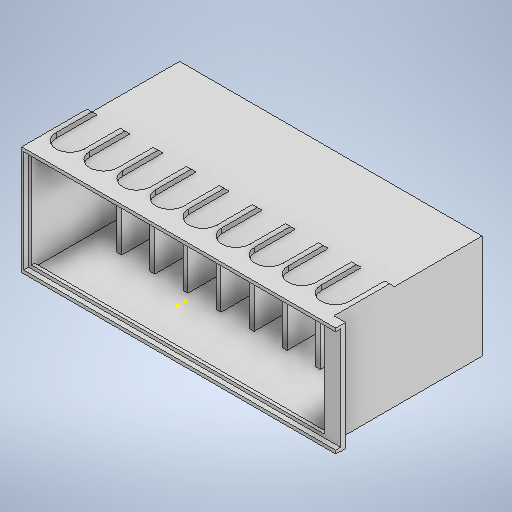
# Autodesk Inventor part: Storage
Saved by Autodesk Inventor 2025.2 (Build 292293000, 293)
## iProperties
Created: 2025-04-05
Part Number: Storage
Material: Generic
Document SubType Name: Modeling
Designer: pipep
Density: 1 g/cm^3
Appearance: Default
Author: pipep
Autodesk Inventor part; units mm, degrees
ref_plane "YZ Plane" through (0, 0, 0) normal (1, 0, 0) x (0, 1, 0)
ref_plane "XZ Plane" through (0, 0, 0) normal (0, 1, 0) x (-1, 0, 0)
ref_plane "XY Plane" through (0, 0, 0) normal (0, 0, 1) x (1, 0, 0)
sketch "Sketch1" plane through (0, 0, 0) normal (0, 0, 1) x (1, 0, 0)
  line L0 (2.6533, -0.0823) -> (-97.3467, -0.0823)
  line L1 (-97.3467, -0.0823) -> (-97.3467, 31.7677)
  line L2 (-97.3467, 31.7677) -> (102.6533, 31.7677)
  line L3 (102.6533, 31.7677) -> (102.6533, -31.9323)
  line L4 (102.6533, -31.9323) -> (-97.3467, -31.9323)
  line L5 (-97.3467, -31.9323) -> (-97.3467, 31.7677)
  point P0 (0, 0)
  dimension "d0" = 100
  dimension "d1" = 31.85
  dimension "d2" = 200
  dimension "d3" = 63.7
  constraints: 12 end point, 2 horizontal, 2 parallel, 2 perpendicular
  measures "d0" distance of L0.start L0.end
  measures "d1" distance of L0.end L1.end
  measures "d2" distance of L3.end L4.end
  measures "d3" distance of L2.end L3.end
extrude "Extrusion1" add sketch "Sketch1" along normal blind 56.62
sketch "Sketch2" plane through (0, 0, 56.62) normal (0, 0, 1) x (1, 0, 0)
  line L0 (-97.3467, 31.7677) -> (-97.3467, -31.9323) projected
  line L1 (-97.3467, -0.0823) -> (-94.3467, -0.0823)
  line L2 (-94.3467, -0.0823) -> (-94.3467, 29.7677)
  line L3 (-94.3467, 29.7677) -> (-77.1067, 29.7677)
  line L4 (102.6533, 31.7677) -> (-97.3467, 31.7677) projected
  line L5 (-94.3467, 29.7677) -> (-77.1067, 29.7677)
  line L6 (-77.1067, 29.7677) -> (-77.1067, -29.9323)
  line L7 (-77.1067, -29.9323) -> (-94.3467, -29.9323)
  line L8 (-94.3467, -29.9323) -> (-94.3467, 29.7677)
  line L9 (-77.1067, -0.0823) -> (-74.1067, -0.0823)
  line L10 (-74.1067, -0.0823) -> (-74.1067, 29.7677)
  line L11 (-74.1067, 29.7677) -> (-56.8667, 29.7677)
  line L12 (-74.1067, 29.7677) -> (-56.8667, 29.7677)
  line L13 (-56.8667, 29.7677) -> (-56.8667, -29.9323)
  line L14 (-56.8667, -29.9323) -> (-74.1067, -29.9323)
  line L15 (-74.1067, -29.9323) -> (-74.1067, 29.7677)
  line L16 (-56.8667, -0.0823) -> (-53.8667, -0.0823)
  line L17 (-53.8667, -0.0823) -> (-53.8667, 29.7677)
  line L18 (-53.8667, 29.7677) -> (-36.6267, 29.7677)
  line L19 (-53.8667, 29.7677) -> (-36.6267, 29.7677)
  line L20 (-36.6267, 29.7677) -> (-36.6267, -29.9323)
  line L21 (-36.6267, -29.9323) -> (-53.8667, -29.9323)
  line L22 (-53.8667, -29.9323) -> (-53.8667, 29.7677)
  line L23 (-36.6267, -0.0823) -> (-33.6267, -0.0823)
  line L24 (-33.6267, -0.0823) -> (-33.6267, 29.7677)
  line L25 (-33.6267, 29.7677) -> (-16.3867, 29.7677)
  line L26 (-33.6267, 29.7677) -> (-16.3867, 29.7677)
  line L27 (-16.3867, 29.7677) -> (-16.3867, -29.9323)
  line L28 (-16.3867, -29.9323) -> (-33.6267, -29.9323)
  line L29 (-33.6267, -29.9323) -> (-33.6267, 29.7677)
  line L30 (-16.3867, -0.0823) -> (-13.3867, -0.0823)
  line L31 (-13.3867, -0.0823) -> (-13.3867, 29.7677)
  line L32 (-13.3867, 29.7677) -> (3.8533, 29.7677)
  line L33 (-13.3867, 29.7677) -> (3.8533, 29.7677)
  line L34 (3.8533, 29.7677) -> (3.8533, -29.9323)
  line L35 (3.8533, -29.9323) -> (-13.3867, -29.9323)
  line L36 (-13.3867, -29.9323) -> (-13.3867, 29.7677)
  line L37 (3.8533, -0.0823) -> (6.8533, -0.0823)
  line L38 (6.8533, -0.0823) -> (6.8533, 29.7677)
  line L39 (6.8533, 29.7677) -> (24.0933, 29.7677)
  line L40 (6.8533, 29.7677) -> (24.0933, 29.7677)
  line L41 (24.0933, 29.7677) -> (24.0933, -29.9323)
  line L42 (24.0933, -29.9323) -> (6.8533, -29.9323)
  line L43 (6.8533, -29.9323) -> (6.8533, 29.7677)
  line L44 (24.0933, -0.0823) -> (27.0933, -0.0823)
  line L45 (27.0933, -0.0823) -> (27.0933, 29.7677)
  line L46 (27.0933, 29.7677) -> (44.3333, 29.7677)
  line L47 (27.0933, 29.7677) -> (44.3333, 29.7677)
  line L48 (44.3333, 29.7677) -> (44.3333, -29.9323)
  line L49 (44.3333, -29.9323) -> (27.0933, -29.9323)
  line L50 (27.0933, -29.9323) -> (27.0933, 29.7677)
  line L51 (64.5733, -0.0823) -> (67.5733, -0.0823)
  line L52 (67.5733, -0.0823) -> (67.5733, 29.7677)
  line L53 (67.5733, 29.7677) -> (84.8133, 29.7677)
  line L54 (67.5733, 29.7677) -> (84.8133, 29.7677)
  line L55 (84.8133, 29.7677) -> (84.8133, -29.9323)
  line L56 (84.8133, -29.9323) -> (67.5733, -29.9323)
  line L57 (67.5733, -29.9323) -> (67.5733, 29.7677)
  line L58 (84.8133, -0.0823) -> (87.8133, -0.0823)
  line L59 (87.8133, -0.0823) -> (87.8133, 29.7677)
  line L60 (87.8133, 29.7677) -> (105.0533, 29.7677)
  line L61 (87.8133, 29.7677) -> (105.0533, 29.7677)
  line L62 (105.0533, 29.7677) -> (105.0533, -29.9323)
  line L63 (105.0533, -29.9323) -> (87.8133, -29.9323)
  line L64 (87.8133, -29.9323) -> (87.8133, 29.7677)
  line L65 (44.3333, -0.0823) -> (47.3333, -0.0823)
  line L66 (47.3333, -0.0823) -> (47.3333, 29.7677)
  line L67 (47.3333, 29.7677) -> (64.5733, 29.7677)
  line L68 (47.3333, 29.7677) -> (64.5733, 29.7677)
  line L69 (64.5733, 29.7677) -> (64.5733, -29.9323)
  line L70 (64.5733, -29.9323) -> (47.3333, -29.9323)
  line L71 (47.3333, -29.9323) -> (47.3333, 29.7677)
  line L72 (87.8133, -35.0469) -> (105.0533, -35.0469)
  line L73 (105.0533, -35.0469) -> (105.0533, 39.0477)
  line L74 (105.0533, 39.0477) -> (87.8133, 39.0477)
  line L75 (87.8133, 39.0477) -> (87.8133, -35.0469)
  point P0 (0, 0)
  dimension "d6" = 3
  dimension "d7" = 29.85
  dimension "d8" = 17.24
  dimension "d9" = 90
  dimension "d10" = 59.7
  dimension "d11" = 3
  dimension "d12" = 29.85
  dimension "d13" = 17.24
  dimension "d14" = 90
  dimension "d15" = 59.7
  dimension "d16" = 3
  dimension "d17" = 29.85
  dimension "d18" = 17.24
  dimension "d19" = 90
  dimension "d20" = 59.7
  dimension "d21" = 3
  dimension "d22" = 29.85
  dimension "d23" = 17.24
  dimension "d24" = 90
  dimension "d25" = 59.7
  dimension "d26" = 3
  dimension "d27" = 29.85
  dimension "d28" = 17.24
  dimension "d29" = 90
  dimension "d30" = 59.7
  dimension "d31" = 3
  dimension "d32" = 29.85
  dimension "d33" = 17.24
  dimension "d34" = 90
  dimension "d35" = 59.7
  dimension "d36" = 3
  dimension "d37" = 29.85
  dimension "d38" = 17.24
  dimension "d39" = 90
  dimension "d40" = 59.7
  dimension "d41" = 3
  dimension "d42" = 29.85
  dimension "d43" = 17.24
  dimension "d44" = 90
  dimension "d45" = 59.7
  dimension "d46" = 3
  dimension "d47" = 29.85
  dimension "d48" = 17.24
  dimension "d49" = 90
  dimension "d50" = 59.7
  dimension "d51" = 3
  dimension "d52" = 29.85
  dimension "d53" = 17.24
  dimension "d54" = 90
  dimension "d55" = 59.7
  constraints: 148 end point, 23 parallel, 21 horizontal, 21 perpendicular, 1 midpoint
  measures "d6" distance of L1.start L1.end
  measures "d7" distance of L1.end L2.end
  measures "d8" distance of L2.end L3.end
  measures "d9" angle of L2 L3
  measures "d10" distance of L5.end L6.end
  measures "d11" distance of L9.start L9.end
  measures "d12" distance of L9.end L10.end
  measures "d13" distance of L10.end L11.end
  measures "d14" angle of L10 L11
  measures "d15" distance of L12.end L13.end
  measures "d16" distance of L16.start L16.end
  measures "d17" distance of L16.end L17.end
  measures "d18" distance of L17.end L18.end
  measures "d19" angle of L17 L18
  measures "d20" distance of L19.end L20.end
  measures "d21" distance of L23.start L23.end
  measures "d22" distance of L23.end L24.end
  measures "d23" distance of L24.end L25.end
  measures "d24" angle of L24 L25
  measures "d25" distance of L26.end L27.end
  measures "d26" distance of L30.start L30.end
  measures "d27" distance of L30.end L31.end
  measures "d28" distance of L31.end L32.end
  measures "d29" angle of L31 L32
  measures "d30" distance of L33.end L34.end
  measures "d31" distance of L37.start L37.end
  measures "d32" distance of L37.end L38.end
  measures "d33" distance of L38.end L39.end
  measures "d34" angle of L38 L39
  measures "d35" distance of L40.end L41.end
  measures "d36" distance of L44.start L44.end
  measures "d37" distance of L44.end L45.end
  measures "d38" distance of L45.end L46.end
  measures "d39" angle of L45 L46
  measures "d40" distance of L47.end L48.end
  measures "d41" distance of L51.start L51.end
  measures "d42" distance of L51.end L52.end
  measures "d43" distance of L52.end L53.end
  measures "d44" angle of L52 L53
  measures "d45" distance of L54.end L55.end
  measures "d46" distance of L58.start L58.end
  measures "d47" distance of L58.end L59.end
  measures "d48" distance of L59.end L60.end
  measures "d49" angle of L59 L60
  measures "d50" distance of L61.end L62.end
  measures "d51" distance of L65.start L65.end
  measures "d52" distance of L65.end L66.end
  measures "d53" distance of L66.end L67.end
  measures "d54" angle of L66 L67
  measures "d55" distance of L68.end L69.end
extrude "Extrusion2" cut sketch "Sketch2" against normal blind 56.62 contours L75 L74 L73 L60 | L2 L3 L6 L7 L8 | L60 L62 L63 L64 L59 | L55 L56 L57 L52 L53 | L63 L73 L72 L75 | L10 L11 L13 L14 L15 | L69 L70 L71 L66 L67 | L17 L18 L20 L21 L22 | L48 L49 L50 L45 L46 | L24 L25 L27 L28 L29 | L41 L42 L43 L38 L39 | L31 L32 L34 L35 L36
sketch "Sketch4" plane through (0, 0, 0) normal (0, 0, -1) x (-1, 0, 0)
  line L0 (-87.8133, 31.7677) -> (-87.8133, -31.9323) projected
  line L1 (97.3467, -31.9323) -> (-87.8133, -31.9323) projected
  line L2 (-87.8133, 31.7677) -> (97.3467, 31.7677)
  line L3 (97.3467, 31.7677) -> (97.3467, -31.9323)
  line L4 (97.3467, -31.9323) -> (-87.8133, -31.9323)
  line L5 (-87.8133, -31.9323) -> (-87.8133, 31.7677)
  point P0 (0, 0)
  constraints: 8 end point, 2 parallel, 1 horizontal, 1 perpendicular
extrude "Extrusion4" add sketch "Sketch4" along normal blind 2
sketch "Sketch5" plane through (0, 0, 56.62) normal (0, 0, 1) x (1, 0, 0)
  line L0 (-94.3467, 29.7677) -> (-94.3467, 34.7677)
  line L1 (-94.3467, 34.7677) -> (-97.3467, 34.7677)
  line L2 (-97.3467, 34.7677) -> (87.8133, 34.7677)
  line L3 (87.8133, 34.7677) -> (87.8133, -31.9323)
  line L4 (87.8133, -31.9323) -> (-97.3467, -31.9323)
  line L5 (-97.3467, -31.9323) -> (-97.3467, 34.7677)
  line L6 (84.8133, 29.7677) -> (84.8133, -29.9323) projected
  line L7 (-94.3467, 29.7677) -> (84.8133, 29.7677)
  line L8 (84.8133, 29.7677) -> (84.8133, -29.9323)
  line L9 (84.8133, -29.9323) -> (-94.3467, -29.9323)
  line L10 (-94.3467, -29.9323) -> (-94.3467, 29.7677)
  point P0 (0, 0)
  dimension "d69" = 5
  dimension "d70" = 3
  constraints: 20 end point, 4 parallel, 3 horizontal, 2 perpendicular, 1 vertical
  measures "d69" distance of L0.start L0.end
  measures "d70" distance of L0.end L1.end
extrude "Extrusion5" add sketch "Sketch5" along normal blind 40 and the other way blind 5
sketch "Sketch11" plane through (87.8133, -31.9323, -2) normal (1, 0, 0) x (0, 0, -1)
  line L0 (-98.62, 66.7) -> (-53.62, 66.7) projected
  line L1 (-98.62, 66.7) -> (-98.62, 64.7)
  line L2 (-98.62, 66.7) -> (-98.62, 0) projected
  line L3 (-98.62, 64.7) -> (-93.62, 64.7)
  line L4 (-98.62, 0) -> (-98.62, 2.6466)
  line L5 (0, 0) -> (-98.62, 0) projected
  line L6 (-98.62, 2) -> (-98.62, 61.7) projected
  line L7 (-98.62, 0) -> (-98.62, 2)
  line L8 (-98.62, 2) -> (-96.62, 2)
  line L9 (-93.62, 64.7) -> (-96.62, 64.7)
  line L10 (-96.62, 64.7) -> (-96.62, 2)
  line L11 (-96.62, 2) -> (-93.62, 2)
  line L12 (-93.62, 2) -> (-93.62, 64.7)
  point P0 (-2, 31.9323)
  dimension "d95" = 2
  dimension "d96" = 5
  dimension "d97" = 2
  dimension "d98" = 2
  constraints: 18 end point, 2 horizontal, 2 parallel, 2 perpendicular, 2 point on line, 1 vertical
  measures "d95" distance of L0.start L1.end
  measures "d96" distance of L1.end L3.end
  measures "d97" distance of L2.end L6.start
  measures "d98" distance of L6.start L8.end
extrude "Extrusion10" cut sketch "Sketch11" against normal blind 184 contours L3 L12 L11 L10
sketch "Sketch12" plane through (-94.3467, -29.9323, 96.62) normal (1, 0, 0) x (0, 0, -1)
  line L0 (0, 0) -> (2, 0) projected
  line L1 (0, 0) -> (0, 3)
  line L2 (0, 0) -> (0, 59.7) projected
  line L3 (0, 3) -> (2, 3)
  line L4 (2, 3) -> (2, 0)
  line L5 (2, 0) -> (0, 0)
  line L6 (5, 0) -> (5, 3)
  line L7 (5, 59.7) -> (5, 0) projected
  line L8 (5, 3) -> (7, 3)
  line L9 (7, 3) -> (7, 0)
  line L10 (5, 0) -> (96.62, 0) projected
  line L11 (7, 0) -> (5, 0)
  point P0 (96.62, 29.9323)
  dimension "d101" = 3
  dimension "d102" = 2
  dimension "d103" = 3
  dimension "d104" = 3
  dimension "d105" = 2
  dimension "d106" = 3
  dimension "d107" = 2
  constraints: 16 end point, 4 point on line, 2 perpendicular
  measures "d101" distance of L0.start L1.end
  measures "d102" distance of L1.end L3.end
  measures "d103" distance of L3.end L4.end
  measures "d104" distance of L6.start L6.end
  measures "d105" distance of L6.end L8.end
  measures "d106" distance of L8.end L9.end
  measures "d107" distance of L9.end L6.start
extrude "Extrusion11" add sketch "Sketch12" along normal blind 180
sketch "Sketch13" plane through (0, 0, 96.62) normal (0, 0, 1) x (1, 0, 0)
  point P0 (0, 0)
sketch "Sketch14" plane through (87.8133, -29.9323, 91.62) normal (0, 0, 1) x (1, 0, 0)
  point P0 (-87.8133, 29.9323)
sketch "Sketch15" plane through (0, 0, 96.62) normal (0, 0, 1) x (1, 0, 0)
  line L0 (87.8133, 34.7677) -> (-97.3467, 34.7677) projected
  line L1 (87.8133, -31.9323) -> (87.8133, 34.7677) projected
  line L2 (-97.3467, 34.7677) -> (87.8133, 34.7677)
  line L3 (87.8133, 34.7677) -> (87.8133, -31.9323)
  line L4 (87.8133, -31.9323) -> (-97.3467, -31.9323)
  line L5 (-97.3467, -31.9323) -> (-97.3467, 34.7677)
  point P0 (0, 0)
  constraints: 8 end point, 2 parallel, 1 horizontal, 1 perpendicular
extrude "Extrusion12" cut sketch "Sketch15" against normal blind 2
sketch "Sketch16" plane through (0, 0, 0) normal (0, 0, 1) x (1, 0, 0)
  point P0 (0, 0)
sketch "Sketch17" plane through (-94.3467, -26.9323, 89.62) normal (0, 1, 0) x (1, 0, 0)
  line L0 (0, 0) -> (179.16, 0) projected
  line L1 (0, 0) -> (179.16, 0)
  line L2 (179.16, 0) -> (179.16, -2)
  line L3 (179.16, -2) -> (0, -2)
  line L4 (0, -2) -> (0, 0)
  point P0 (94.3467, 89.62)
  constraints: 8 end point, 2 parallel, 1 horizontal, 1 perpendicular
extrude "Extrusion13" cut sketch "Sketch17" against normal blind 1
sketch "Sketch18" plane through (-97.3467, 34.7677, 51.62) normal (0, 1, 0) x (1, 0, 0)
  line L0 (185.16, 0) -> (182.16, 0)
  line L1 (0, -43) -> (0, 0) projected
  line L2 (0, 0) -> (3, 0)
  line L3 (3, -40) -> (3, 51.62) projected
  line L4 (3, 0) -> (3, -25)
  line L5 (185.16, -43) -> (1.16, -43) projected
  arc A0 (3, -25) -> (20.24, -25) centre (11.62, -25) ccw
  line L6 (3, 0) -> (20.24, 0)
  line L7 (20.24, 0) -> (20.24, -25)
  line L8 (3, -25) -> (3, 0)
  line L9 (23.24, 0.3271) -> (23.24, -24.6729)
  arc A1 (23.24, -24.6729) -> (40.48, -24.6729) centre (31.86, -24.6729) ccw
  line L10 (40.48, 0.3271) -> (40.48, -24.6729)
  line L11 (23.24, -24.6729) -> (23.24, 0.3271)
  line L12 (43.48, 0.3271) -> (43.48, -24.6729)
  arc A2 (43.48, -24.6729) -> (60.72, -24.6729) centre (52.1, -24.6729) ccw
  line L13 (60.72, 0.3271) -> (60.72, -24.6729)
  line L14 (43.48, -24.6729) -> (43.48, 0.3271)
  line L15 (63.72, 0.3271) -> (63.72, -24.6729)
  arc A3 (63.72, -24.6729) -> (80.96, -24.6729) centre (72.34, -24.6729) ccw
  line L16 (80.96, 0.3271) -> (80.96, -24.6729)
  line L17 (63.72, -24.6729) -> (63.72, 0.3271)
  line L18 (83.96, 0.3271) -> (83.96, -24.6729)
  arc A4 (83.96, -24.6729) -> (101.2, -24.6729) centre (92.58, -24.6729) ccw
  line L19 (101.2, 0.3271) -> (101.2, -24.6729)
  line L20 (83.96, -24.6729) -> (83.96, 0.3271)
  line L21 (104.2, 0.3271) -> (104.2, -24.6729)
  arc A5 (104.2, -24.6729) -> (121.44, -24.6729) centre (112.82, -24.6729) ccw
  line L22 (121.44, 0.3271) -> (121.44, -24.6729)
  line L23 (104.2, -24.6729) -> (104.2, 0.3271)
  line L24 (124.44, 0.3271) -> (124.44, -24.6729)
  arc A6 (124.44, -24.6729) -> (141.68, -24.6729) centre (133.06, -24.6729) ccw
  line L25 (141.68, 0.3271) -> (141.68, -24.6729)
  line L26 (124.44, -24.6729) -> (124.44, 0.3271)
  line L27 (144.68, 0.3271) -> (144.68, -24.6729)
  arc A7 (144.68, -24.6729) -> (161.92, -24.6729) centre (153.3, -24.6729) ccw
  line L28 (161.92, 0.3271) -> (161.92, -24.6729)
  line L29 (144.68, -24.6729) -> (144.68, 0.3271)
  line L30 (164.92, 0.3271) -> (164.92, -24.6729)
  arc A8 (164.92, -24.6729) -> (182.16, -24.6729) centre (173.54, -24.6729) ccw
  line L31 (182.16, 0) -> (182.16, -24.6729)
  line L32 (164.92, -24.6729) -> (164.92, 0.3271)
  line L33 (20.24, 0) -> (182.16, 0)
  line L34 (0, 0) -> (185.16, 0) projected
  point P0 (97.3467, 51.62)
  point P1 (3, -25)
  point P2 (161.92, 0)
  point P3 (144.68, 0)
  point P4 (40.48, 0)
  point P5 (23.24, 0)
  point P6 (141.68, 0)
  point P7 (124.44, 0)
  point P8 (60.72, 0)
  point P9 (43.48, 0)
  point P10 (121.44, 0)
  point P11 (104.2, 0)
  point P12 (80.96, 0)
  point P13 (63.72, 0)
  point P14 (101.2, 0)
  point P15 (83.96, 0)
  point P16 (164.92, 0)
  dimension "d115" = 3
  dimension "d119" = 3
  dimension "d120" = 25
  dimension "d121" = 17.24
  dimension "d122" = 25
  dimension "d123" = 17.24
  dimension "d124" = 25
  dimension "d125" = 17.24
  dimension "d126" = 25
  dimension "d127" = 17.24
  dimension "d128" = 25
  dimension "d129" = 17.24
  dimension "d130" = 25
  dimension "d131" = 17.24
  dimension "d132" = 25
  dimension "d133" = 17.24
  dimension "d134" = 25
  dimension "d135" = 17.24
  dimension "d138" = 25
  dimension "d139" = 17.24
  constraints: 62 end point, 18 point on circle, 9 centre point, 9 parallel, 9 tangent, 2 perpendicular, 1 collinear, 1 horizontal, 1 point on line
  measures "d115" distance of L0.start L0.end
  measures "d119" distance of L1.end L2.end
  measures "d120" distance of L2.end L4.end
  measures "d121" distance of L4.end L7.end
  measures "d122" distance of L9.start L9.end
  measures "d123" distance of L9.end L10.end
  measures "d124" distance of L12.start L12.end
  measures "d125" distance of L12.end L13.end
  measures "d126" distance of L15.start L15.end
  measures "d127" distance of L15.end L16.end
  measures "d128" distance of L18.start L18.end
  measures "d129" distance of L18.end L19.end
  measures "d130" distance of L21.start L21.end
  measures "d131" distance of L21.end L22.end
  measures "d132" distance of L24.start L24.end
  measures "d133" distance of L24.end L25.end
  measures "d134" distance of L27.start L27.end
  measures "d135" distance of L27.end L28.end
  measures "d138" distance of L30.start L30.end
  measures "d139" distance of L30.end L31.end
extrude "Extrusion14" cut sketch "Sketch18" against normal blind 3
chamfer "Chamfer1" distance 3 angle 45 10 edges at (-95.8467, 34.7677, 51.62) (-75.6067, 34.7677, 51.62) (-55.3667, 34.7677, 51.62) (-35.1267, 34.7677, 51.62) (-14.8867, 34.7677, 51.62) (5.3533, 34.7677, 51.62) (25.5933, 34.7677, 51.62) (45.8333, 34.7677, 51.62) (66.0733, 34.7677, 51.62) (86.3133, 34.7677, 51.62)
sketch "Sketch19" plane through (-94.3467, 29.7677, 0) normal (0, -1, 0) x (1, 0, 0)
  point P0 (94.3467, 0)
sketch "Sketch20" plane through (-94.3467, 29.7677, 0) normal (0, -1, 0) x (1, 0, 0)
  point P0 (94.3467, 0)
sketch "Sketch21" plane through (0, 0, -2) normal (0, 0, -1) x (-1, 0, 0)
  point P0 (0, 0)
sketch "Sketch22" plane through (87.8133, -31.9323, -2) normal (1, 0, 0) x (0, 0, -1)
  line L0 (0, 0) -> (-96.62, 0)
  line L1 (-96.62, 66.7) -> (-56.62, 66.7) projected
  line L2 (-96.62, 0) -> (-96.62, 66.7)
  line L3 (-96.62, 66.7) -> (-93.62, 66.7)
  line L4 (-93.62, 66.7) -> (-93.62, 0)
  line L5 (-96.62, 66.7) -> (-93.62, 66.7)
  line L6 (-93.62, 66.7) -> (-93.62, 64.7)
  line L7 (-93.62, 64.7) -> (-96.62, 64.7)
  line L8 (-96.62, 64.7) -> (-96.62, 66.7)
  line L9 (-96.62, 0) -> (-93.62, 0)
  line L10 (-93.62, 0) -> (-93.62, 2)
  line L11 (-93.62, 2) -> (-96.62, 2)
  line L12 (-96.62, 2) -> (-96.62, 0)
  line L13 (-93.62, 66.7) -> (-90.62, 66.7)
  line L14 (-90.62, 66.7) -> (-90.62, -0.2532)
  line L15 (-90.62, -0.2532) -> (-93.62, -0.2532)
  line L16 (-93.62, -0.2532) -> (-93.62, 66.7)
  point P0 (-2, 31.9323)
  point P1 (-93.62, 2)
  point P2 (-96.62, 2)
  dimension "d148" = 3
  dimension "d149" = 3
  dimension "d150" = 2
  dimension "d151" = 3
  dimension "d152" = 2
  dimension "d153" = 3
  constraints: 32 end point, 6 parallel, 5 perpendicular, 3 horizontal, 2 point on line
  measures "d148" distance of L1.start L3.end
  measures "d149" distance of L6.end L7.end
  measures "d150" distance of L5.end L6.end
  measures "d151" distance of L11.end L10.end
  measures "d152" distance of L10.end L9.end
  measures "d153" distance of L14.end L15.end
extrude "Extrusion15" add sketch "Sketch22" along normal blind 7 contours L4 L1 L14 L0 | L0 L2 L11 L4 | L0 L14 L15 L16 | L7 L2 L1 L4
sketch "Sketch6" plane through (87.8133, -31.9323, -2) normal (1, 0, 0) x (0, 0, -1)
  line L0 (-98.62, 0) -> (-98.62, 66.7) projected
  line L1 (-98.62, 66.7) -> (-98.62, 64.7)
  line L2 (-98.62, 64.7) -> (-93.62, 64.7)
  line L3 (-98.62, 0) -> (0, 0) projected
  line L4 (-98.62, 0) -> (-98.62, 2)
  line L5 (-98.62, 2) -> (-96.62, 2)
  line L6 (-93.62, 64.7) -> (-96.62, 64.7)
  line L7 (-96.62, 64.7) -> (-96.62, 2)
  line L8 (-96.62, 2) -> (-93.62, 2)
  line L9 (-93.62, 2) -> (-93.62, 64.7)
  point P0 (-2, 31.9323)
  dimension "d75" = 2
  dimension "d76" = 5
  dimension "d77" = 2
  dimension "d78" = 2
  constraints: 16 end point, 3 perpendicular, 2 parallel, 2 point on line, 1 horizontal
  measures "d75" distance of L0.end L1.end
  measures "d76" distance of L1.end L2.end
  measures "d77" distance of L0.start L4.end
  measures "d78" distance of L4.end L5.end
sketch "Sketch7" plane through (-94.3467, -29.9323, 96.62) normal (1, 0, 0) x (0, 0, -1)
  line L0 (0, 0) -> (0, 3)
  line L1 (0, 0) -> (0, 59.7) projected
  line L2 (0, 3) -> (2, 3)
  line L3 (2, 3) -> (2, 0)
  line L4 (2, 0) -> (0, 0)
  line L5 (5, 59.7) -> (5, 0) projected
  line L6 (5, 0) -> (5, 3)
  line L7 (5, 3) -> (7, 3)
  line L8 (7, 3) -> (7, 0)
  line L9 (7, 0) -> (5, 0)
  point P0 (96.62, 29.9323)
  dimension "d81" = 3
  dimension "d82" = 2
  dimension "d83" = 3
  dimension "d84" = 2
  dimension "d85" = 3
  constraints: 16 end point, 4 point on line, 3 perpendicular
  measures "d81" distance of L0.start L0.end
  measures "d82" distance of L0.end L2.end
  measures "d83" distance of L5.end L6.end
  measures "d84" distance of L6.end L7.end
  measures "d85" distance of L7.end L8.end
sketch "Sketch8" plane through (0, 0, 96.62) normal (0, 0, 1) x (1, 0, 0)
  line L0 (87.8133, 34.7677) -> (-97.3467, 34.7677) projected
  line L1 (-97.3467, 34.7677) -> (-97.3467, 36.7677)
  line L2 (87.8133, 34.7677) -> (87.8133, 36.7677)
  line L3 (-97.3467, 36.7677) -> (87.8133, 36.7677)
  line L4 (-97.3467, -31.9323) -> (87.8133, -31.9323) projected
  line L5 (-97.3467, 34.7677) -> (87.8133, 34.7677)
  line L6 (87.8133, 34.7677) -> (87.8133, -31.9323)
  line L7 (87.8133, -31.9323) -> (-97.3467, -31.9323)
  line L8 (-97.3467, -31.9323) -> (-97.3467, 34.7677)
  point P0 (0, 0)
  dimension "d88" = 2
  dimension "d89" = 2
  dimension "d90" = 185.16
  constraints: 14 end point, 2 parallel, 2 vertical, 1 horizontal, 1 perpendicular
  measures "d88" distance of L0.end L1.end
  measures "d89" distance of L0.start L2.end
  measures "d90" distance of L1.end L2.end
sketch "Sketch9" plane through (87.8133, -29.9323, 91.62) normal (0, 0, 1) x (1, 0, 0)
  line L0 (-3, 0) -> (-3, 3) projected
  line L1 (0, 0) -> (-3, 0)
  line L2 (-3, 0) -> (-3, 3)
  line L3 (-3, 3) -> (0, 3)
  line L4 (0, 3) -> (0, 0)
  line L5 (-182.16, 3) -> (-3, 3) projected
  line L6 (-182.16, 3) -> (-185.16, 3)
  line L7 (-185.16, 0) -> (-185.16, 62.7) projected
  line L8 (0, 0) -> (-185.16, 0) projected
  line L9 (-185.16, 0) -> (-182.16, 0)
  line L10 (-182.16, 0) -> (-182.16, 3)
  line L11 (-182.16, 3) -> (-185.16, 3)
  line L12 (-185.16, 3) -> (-185.16, 0)
  line L13 (-3, 3) -> (0, 3)
  line L14 (0, 3) -> (0, 0)
  line L15 (0, 0) -> (-3, 0)
  line L16 (-3, 0) -> (-3, 3)
  point P0 (-87.8133, 29.9323)
  constraints: 26 end point, 6 parallel, 4 horizontal, 3 perpendicular, 1 point on line
equation "\"d2\" = 2 * d0"
equation "\"d3\" = 2 * d1"
body "Solid1"
